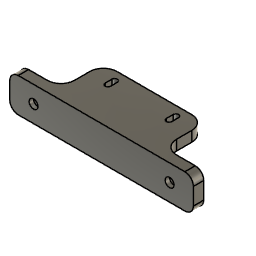
tool_holder_parking_syringe_pump v5 (Autodesk Fusion 360 design; units mm, degrees)
Autodesk Fusion 360 part; units mm, degrees
note: some values were not read from the file. Set by a fixed rule: which sketch regions a step uses.
sketch "Sketch1" plane through (0, 0, 0) normal (0, 1, 0) x (1, 0, 0)
  line L0 (0, 0) -> (0, -20)
  line L1 (0, -20) -> (54, -20)
  line L2 (54, -20) -> (54, 0)
  line L3 (54, 0) -> (0, 0)
  line L4 (0, -20) -> (-54, -20)
  line L5 (-54, -20) -> (-54, 0)
  line L6 (-54, 0) -> (0, 0)
  line L7 (54, 0) -> (54, -14)
  line L8 (54, -14) -> (40, -14)
  line L9 (40, -14) -> (40, -10)
  circle A0 centre (40, -10) radius 5
  line L10 (0, -20) -> (30, -20)
  line L11 (30, -20) -> (30, -14)
  line L12 (30, -14) -> (0, -14)
  line L13 (0, -14) -> (2.72, -14)
  line L14 (0, -14) -> (0, -3.5)
  line L15 (2.72, -14) -> (6.4973, -3.622)
  line L16 (2.72, -14) -> (13.7641, -14) construction
  line L17 (6.4973, -3.622) -> (0, -3.5)
  line L18 (-30, -14) -> (0, -14)
  line L19 (-30, -20) -> (-30, -14)
  line L20 (0, -20) -> (-30, -20)
  line L21 (-2.72, -14) -> (-6.4973, -3.622)
  line L22 (-6.4973, -3.622) -> (0, -3.5)
  circle A1 centre (-40, -10) radius 5
  dimension "d1" = 20
  dimension "d2" = 54
  dimension "d3" = 14
  dimension "d4" = 14
  dimension "d5" = 10
  dimension "d6" = 30
  dimension "d7" = 6
  dimension "d8" = 2.72
  dimension "d9" = 10.5
  dimension "d10" = 70
  dimension "d39" = 6.4973
  constraint coincident L0.start L3.end
  constraint vertical L0
  constraint perpendicular L0 L1
  constraint perpendicular L1 L2
  constraint perpendicular L0 L3
  constraint symmetric L1.start L0 L4.start
  constraint symmetric L0 L1.end L4.end
  constraint symmetric L0 L2.end L5.end
  constraint symmetric L0 L3.end L6.end
  constraint perpendicular L3 L7
  constraint perpendicular L7 L8
  constraint perpendicular L8 L9
  constraint coincident L9.end A0.centre
  constraint perpendicular L0 L10
  constraint perpendicular L1 L11
  constraint coincident L0 L12.end
  constraint perpendicular L0 L12
  constraint perpendicular L0 L13
  constraint perpendicular L13 L14
  constraint horizontal L16
  constraint symmetric L0 L1.start L4.start
  constraint symmetric L0 A0 A1
  constraint symmetric L0 L10.end L19.start
  constraint symmetric L0 L11.end L18.start
  constraint symmetric L0 L12.end L13.start
  constraint symmetric L0 L13.end L21.start
  constraint symmetric L0 L14.end L17.end
  constraint symmetric L0 L15.end L21.end
  measures "d1" distance of L0.start L0.end
  measures "d2" distance of L0.end L1.end
  measures "d3" distance of L2.end L7.end
  measures "d4" distance of L7.end L8.end
  measures "d5" diameter of A0
  measures "d6" distance of L0.end L10.end
  measures "d7" distance of L10.end L11.end
  measures "d8" distance of L12.end L13.end
  measures "d9" distance of L12.end L14.end
  measures "d10" angle of L15 L16
  measures "d39" horizontal distance of L14.end L15.end
extrude "Extrude1" add sketch "Sketch1" along normal blind 25 contours L0 L1 L10 L11 L12 L13 | L0 L4 L18 L19 L20
extrude "Extrude2" add sketch "Sketch1" along normal blind 19 contours L0 L12 L13 L14 L15 L17 | L0 L14 L18 L21 L22
extrude "Extrude3" add sketch "Sketch1" against normal blind 6.1
sketch "Sketch2" plane through (0, -6.1, 0) normal (0, -1, 0) x (1, 0, 0)
  circle A0 centre (-40, 10) radius 5
  circle A1 centre (40, 10) radius 5
  line L0 (54, 20) -> (-54, 20)
  line L1 (-54, 20) -> (-54, 0)
  line L2 (-54, 0) -> (54, 0)
  line L3 (54, 0) -> (54, 20)
  circle A2 centre (40, 10) radius 2.625
  circle A3 centre (-40, 10) radius 2.625
  dimension "d19" = 5.25
  dimension "d20" = 5.25
  constraint concentric A1 A2
  constraint concentric A0 A3
  measures "d19" diameter of A2
  measures "d20" diameter of A3
sketch "Sketch3" plane through (0, 0, 20) normal (0, 0, 1) x (-1, 0, 0)
  line L0 (-30, 0) -> (-30, -25)
  line L1 (-30, -25) -> (30, -25)
  line L2 (30, -25) -> (30, 0)
  line L3 (30, 0) -> (54, 0)
  line L4 (54, 0) -> (54, 6.1)
  line L5 (54, 6.1) -> (-54, 6.1)
  line L6 (-54, 6.1) -> (-54, 0)
  line L7 (-54, 0) -> (-30, 0)
  line L8 (0, -25) -> (-18, -25)
  line L9 (-16.4, -17.6) -> (-16.4, -19.6)
  line L10 (-16.4, -17.6) -> (-16.4, -15.6)
  line L11 (-19.6, -19.6) -> (-19.6, -15.6)
  circle A0 centre (-18, -19.6) radius 1.6
  circle A1 centre (-18, -15.6) radius 1.6
  line L12 (0, -25) -> (0, 0)
  circle A2 centre (18, -19.6) radius 1.6
  line L13 (16.4, -17.6) -> (16.4, -19.6)
  line L14 (16.4, -17.6) -> (16.4, -15.6)
  line L15 (19.6, -19.6) -> (19.6, -15.6)
  circle A3 centre (18, -15.6) radius 1.6
  dimension "d40" = 18
  dimension "d43" = 2
  dimension "d44" = 2
  dimension "d45" = 3.2
  dimension "d46" = 4
  dimension "d47" = 3.2
  dimension "d48" = 3.2
  constraint midpoint L1 L8.start
  constraint parallel L1 L8
  constraint perpendicular L1 L9
  constraint coincident L12.end origin
  constraint symmetric L9.start L12 L13.start
  constraint symmetric L9.end L12 L13.end
  constraint symmetric L10.end L12 L14.end
  constraint symmetric L11.start L12 L15.start
  constraint symmetric L11.end L12 L15.end
  constraint symmetric A0 L12 A2
  constraint symmetric A1 L12 A3
  measures "d40" distance of L8.start L8.end
  measures "d43" distance of L9.start L9.end
  measures "d44" distance of L9.start L10.end
  measures "d45" distance of L9.end L11.start
  measures "d46" distance of L11.start L11.end
  measures "d47" diameter of A0
  measures "d48" diameter of A1
extrude "Extrude5" cut sketch "Sketch3" against normal blind 6 contours L9 L10 L11 A0 A1 | A0 | A1 | A2 | A2 L13 L14 L15 A3 | A3
extrude "Extrude4" add sketch "Sketch2" against normal blind 2.6 contours A0 | A1
fillet "Fillet1" radius 8 2 edges at (30, 0, 17) (-30, 0, 17)
fillet "Fillet2" radius 8 2 edges at (30, 25, 17) (-30, 25, 17)
fillet "Fillet3" radius 5 4 edges at (-54, -3.05, 0) (54, -3.05, 0) (54, -3.05, 20) (-54, -3.05, 20)
fillet "Fillet4" radius 1 2 edges at (-6.4973, 9.5, 3.622) (6.4973, 9.5, 3.622)
